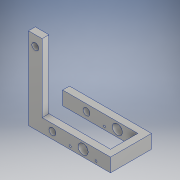
# Autodesk Inventor part: shooter
Saved by Autodesk Inventor 2019 (Build 230136000, 136)
## iProperties
Created: 2019-04-02
Part Number: shooter
Material: Aluminum 6061
Document SubType Name: Modeling
Designer: User
Density: 2.7 g/cm^3
Appearance: Aluminum - Flat
Mass: 367.89 g
Surface Area: 375.999 cm^2
Volume: 136.256 cm^3
Author: User
Autodesk Inventor part; units mm, degrees
ref_plane "YZ Plane" through (0, 0, 0) normal (1, 0, 0) x (0, 1, 0)
ref_plane "XZ Plane" through (0, 0, 0) normal (0, 1, 0) x (-1, 0, 0)
ref_plane "XY Plane" through (0, 0, 0) normal (0, 0, 1) x (1, 0, 0)
sketch "Sketch1" plane through (0, 0, 0) normal (1, 0, 0) x (0, 1, 0)
  line L0 (0, 0) -> (-152.4, 0)
  line L1 (-152.4, 0) -> (-152.4, -12.7)
  line L2 (-152.4, -12.7) -> (0, -12.7)
  line L3 (0, -12.7) -> (0, 0)
  line L4 (0, -12.7) -> (-12.7, -12.7)
  line L5 (-12.7, -63.5) -> (0, -63.5)
  line L6 (0, -63.5) -> (-152.4, -63.5)
  line L7 (-152.4, -63.5) -> (-152.4, -76.2)
  line L8 (-152.4, -76.2) -> (0, -76.2)
  line L9 (0, -76.2) -> (0, -63.5)
  line L10 (-152.4, 0) -> (-139.7, 0)
  line L11 (-139.7, 0) -> (-139.7, -76.2)
  line L12 (-139.7, -76.2) -> (-152.4, -76.2)
  line L13 (-152.4, -76.2) -> (-152.4, 0)
  dimension "d1" = 12.7
  dimension "d4" = 12.7
  dimension "d63" = 12.7
  dimension "d64" = 152.4
  dimension "d65" = 152.4
  dimension "d66" = 50.8
  constraints: 28 end point, 7 parallel, 4 horizontal, 3 perpendicular, 1 collinear, 1 point on line
  measures "d1" distance of L1.end L0.end
  measures "d4" distance of L6.end L7.end
  measures "d63" distance between parallel lines of L13 L11
  measures "d64" distance between parallel lines of L3 L1
  measures "d65" distance between parallel lines of L13 L9
  measures "d66" distance between parallel lines of L6 L2
extrude "Extrusion1" add sketch "Sketch1" along normal blind 25.4
sketch "Sketch2" plane through (0, -152.4, -76.2) normal (0, 0, -1) x (-1, 0, 0)
  line L0 (0, 152.4) -> (-25.4, 152.4) projected
  line L1 (-25.4, 0) -> (-25.4, 152.4) projected
  point P0 (-12.7, 107.95)
  dimension "d8" = 44.45
  dimension "d9" = 25.4
  dimension "d10" = 12.7
  measures "d8" distance from line of L0 point (-12.7, 107.95)
  measures "d9" distance of L0.start L0.end
  measures "d10" distance from line of L1 point (-12.7, 107.95)
hole "Hole1" at (12.7, -44.45, -76.2) direction (0, 0, 1) diameter 12.7 end through all
sketch "Sketch3" plane through (0, -152.4, -76.2) normal (0, 0, -1) x (-1, 0, 0)
  circle A0 centre (-12.7, 107.95) radius 6.35 projected
  line L0 (0, 0) -> (0, 152.4) projected
  line L1 (0, 152.4) -> (-25.4, 152.4) projected
  line L2 (-25.4, 0) -> (-25.4, 152.4) projected
  line L3 (0, 0) -> (-25.4, 0) projected
  point P0 (-12.7, 50.8)
  dimension "d18" = 25.4
  dimension "d19" = 12.7
  dimension "d20" = 50.8
  measures "d18" distance of L0.start L2.start
  measures "d19" distance from line of L2 point (-12.7, 50.8)
  measures "d20" distance from line of L3 point (-12.7, 50.8)
hole "Hole2" at (12.7, -101.6, -76.2) direction (0, 0, 1) diameter 18.4912 end through all
sketch "Sketch4" plane through (0, -152.4, -76.2) normal (0, 0, -1) x (-1, 0, 0)
  circle A0 centre (-12.7, 50.8) radius 9.2456 projected
  circle A1 centre (-12.7, 107.95) radius 6.35 projected
  line L0 (0, 0) -> (0, 152.4) projected
  line L1 (0, 152.4) -> (-25.4, 152.4) projected
  line L2 (-25.4, 0) -> (-25.4, 152.4) projected
  line L3 (0, 0) -> (-25.4, 0) projected
  point P0 (-5.6896, 26.797)
  point P1 (-5.6896, 74.803)
  dimension "d28" = 48.006
  dimension "d29" = 7.0104
  dimension "d30" = 7.0104
  dimension "d31" = 24.003
  measures "d28" distance of point (-5.69, 26.797) point (-5.69, 74.803)
  measures "d29" horizontal distance of point (-5.69, 74.803) A0.centre
  measures "d30" horizontal distance of A0.centre point (-5.69, 26.797)
  measures "d31" vertical distance of A0.centre point (-5.69, 26.797)
hole "Hole3" at (5.6896, -125.603, -76.2) at (5.6896, -77.597, -76.2) direction (0, 0, 1) diameter 3.7084 end through all
sketch "Sketch5" plane through (25.4, 0, 0) normal (1, 0, 0) x (0, 0, -1)
  line L0 (0, 0) -> (12.7, 0)
  line L1 (12.7, 0) -> (12.7, -25.4)
  line L2 (12.7, -25.4) -> (0, -25.4)
  line L3 (0, -25.4) -> (0, 0)
  line L4 (0, 0) -> (0, -152.4) projected
  line L5 (12.7, 0) -> (0, 0) projected
  dimension "d39" = 12.7
  dimension "d67" = 25.4
  dimension "d68" = 0
  dimension "d69" = 0
  constraints: 8 end point, 2 parallel, 1 horizontal, 1 perpendicular
  measures "d39" distance of L1.end L2.end
  measures "d67" distance between parallel lines of L2 L0
  measures "d68" distance between parallel lines of L5 L0
  measures "d69" distance between parallel lines of L3 L4
extrude "Extrusion2" add sketch "Sketch5" along normal blind 127
sketch "Sketch8" plane through (0, -139.7, -12.7) normal (0, 0, -1) x (-1, 0, 0)
  line L0 (-152.4, 114.3) -> (-152.4, 139.7) projected
  line L1 (0, 139.7) -> (-152.4, 139.7) projected
  point P0 (-133.35, 127)
  dimension "d70" = 19.05
  dimension "d71" = 25.4
  dimension "d72" = 12.7
  measures "d70" distance from line of L0 point (-133.35, 127)
  measures "d71" distance of L0.start L0.end
  measures "d72" distance from line of L1 point (-133.35, 127)
hole "Hole6" at (133.35, -12.7, -12.7) direction (0, 0, 1) diameter 12.7 end through all
equation "\"d4\" = d1"
equation "\"d65\" = d64"
equation "\"d10\" = 0.5 * d9"
equation "\"d19\" = 0.5 * d18"
equation "\"d30\" = d29"
equation "\"d31\" = 0.5 * d28"
equation "\"d72\" = 0.5 * d71"
body "Solid1"
